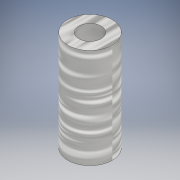
# Autodesk Inventor part: スペーサーm4,18
Saved by Autodesk Inventor 2019.2 (Build 232265000, 265)
## iProperties
Part Number: スペーサーm4,18
Material: アルミニウム 7075
Document SubType Name: Modeling
Designer: 雪村
Density: 2.81 g/cm^3
Appearance: サテン - ブラシ仕上げ 重厚
Mass: 1.90682 g
Surface Area: 7.53982 cm^2
Volume: 0.678584 cm^3
Author: 雪村
Autodesk Inventor part; units mm, degrees
ref_plane "YZ Plane" through (0, 0, 0) normal (1, 0, 0) x (0, 1, 0)
ref_plane "XZ Plane" through (0, 0, 0) normal (0, 1, 0) x (-1, 0, 0)
ref_plane "XY Plane" through (0, 0, 0) normal (0, 0, 1) x (1, 0, 0)
sketch "スケッチ1" plane through (0, 0, 0) normal (0, 0, 1) x (1, 0, 0)
  circle A0 centre (0, 0) radius 2
  circle A1 centre (0, 0) radius 4
  dimension "d0" = 4
  dimension "d1" = 8
  constraints: 2 centre point, 2 coincident
  measures "d0" diameter of A0
  measures "d1" diameter of A1
extrude "押し出し1" add sketch "スケッチ1" along normal blind 18
